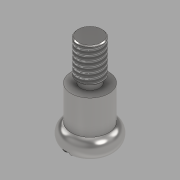
# Autodesk Inventor part: Crank Screw
Saved by Autodesk Inventor 2020 (Build 240168000, 168)
## iProperties
Created: 2019-11-25
Part Number: Crank Screw
Material: Acero inoxidable
Document SubType Name: Modeling
Designer: Gerardo Naranjo
Density: 8 g/cm^3
Appearance: Semipulido
Engineer: Gerardo Naranjo
Author: Gerardo Daniel Naranjo Gallegos
Title: Crank Screw
Autodesk Inventor part; units mm, degrees
ref_plane "YZ Plane" through (0, 0, 0) normal (1, 0, 0) x (0, 1, 0)
ref_plane "XZ Plane" through (0, 0, 0) normal (0, 1, 0) x (-1, 0, 0)
ref_plane "XY Plane" through (0, 0, 0) normal (0, 0, 1) x (1, 0, 0)
sketch "Boceto1" plane through (0, 0, 0) normal (0, 0, 1) x (1, 0, 0)
  line L0 (0, 0) -> (-1.5875, 0)
  line L1 (-1.4605, 11.9062) -> (0, 11.9062)
  line L2 (0, 11.9062) -> (0, 0)
  line L3 (-1.4605, 11.9062) -> (-1.5875, 11.7793)
  line L4 (-1.1906, 7.5375) -> (-1.1906, 6.7437)
  line L5 (-1.4605, 7.5375) -> (-1.1906, 7.5375)
  line L6 (-1.5875, 7.6645) -> (-1.5875, 11.7793)
  line L7 (-1.5875, 7.6645) -> (-1.4605, 7.5375)
  line L8 (0, 0) -> (-1.905, 0)
  line L9 (-2.3813, 6.7469) -> (-1.1906, 6.7469)
  line L10 (0, 6.7469) -> (0, 0)
  arc A0 (-2.3813, 2.4473) -> (-1.905, 0) centre (-1.905, 1.27) ccw
  line L11 (-2.3813, 0) -> (-2.3813, 0.0927)
  line L12 (-2.3813, 2.4473) -> (-2.3813, 6.7469)
  point P0 (-1.5875, 11.9062)
  point P1 (-1.5875, 7.5375)
  dimension "d0" = 1.5875
  dimension "d1" = 11.9062
  dimension "d2" = 0.127
  dimension "d3" = 0.127
  dimension "d5" = 0.7937
  dimension "d7" = 4.3688
  dimension "d8" = 0.127
  dimension "d9" = 0.127
  dimension "d10" = 2.3813
  dimension "d11" = 6.7469
  dimension "d12" = 2.54
  dimension "d13" = 1.27
  dimension "d14" = 1.905
  constraints: 26 end point, 5 parallel, 4 point on line, 3 horizontal, 3 perpendicular, 3 point on circle, 1 centre point, 1 vertical
  measures "d0" distance of point (-1.587, 11.906) L1.end
  measures "d1" distance of L0.end point (-1.587, 11.906)
  measures "d2" distance of L1.start point (-1.587, 11.906)
  measures "d3" distance of L3.end point (-1.587, 11.906)
  measures "d5" distance of L4.start L4.end
  measures "d7" distance from line of L4.start L1
  measures "d8" distance of L6.start point (-1.587, 7.537)
  measures "d9" distance of L5.start point (-1.587, 7.537)
  measures "d10" distance of L9.start L10.start
  measures "d11" distance of L11.start L9.start
  measures "d12" diameter of A0
  measures "d13" distance from line of L0 A0.centre
  measures "d14" distance from line of L2 A0.centre
revolve "Revolución1" add sketch "Boceto1" angle 360 about axis through (0, 11.9062, 0) along (0, -1, 0)
thread "Rosca1" size "5-40 UNC" class "2A" standard "ANSI Unified Screw Threads" full length
sketch "Boceto2" plane through (0, 0, 0) normal (0, -1, 0) x (1, 0, 0)
  line L0 (-0.3969, 3.9709) -> (0.3969, 3.9709)
  line L1 (0.3969, 3.9709) -> (0.3969, -4.5285)
  line L2 (0.3969, -4.5285) -> (-0.3969, -4.5285)
  line L3 (-0.3969, -4.5285) -> (-0.3969, 3.9709)
  point P0 (0, 0)
  dimension "d18" = 0.7937
  dimension "d19" = 0.3969
  constraints: 8 end point, 2 parallel, 1 horizontal, 1 perpendicular
  measures "d18" distance of L1.end L2.end
  measures "d19" distance from line of point (0, 0) L1
extrude "Extrusión1" cut sketch "Boceto2" against normal blind 0.7937
equation "\"d3\" = d2"
equation "\"d7\" = d4"
equation "\"d9\" = d8"
equation "\"d19\" = 0.5 * d18"
equation "\"d4\" = 4.3688"
